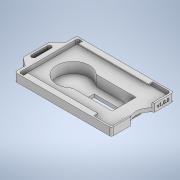
# Autodesk Inventor part: badge
Saved by Autodesk Inventor 2020 (Build 240168000, 168)
## iProperties
Created: 2019-12-22
Part Number: badge
Material: Generic
Document SubType Name: Modeling
Designer: user
Density: 1 g/cm^3
Appearance: Default
Author: user
## iProperties of the stored document _3DPrint.ipt
Created: 2019-12-23
Part Number: _3DPrint
Material: Generic
Document SubType Name: Modeling
Designer: user
Density: 1 g/cm^3
Appearance: Default
Author: user
Autodesk Inventor part; units mm, degrees
ref_plane "YZ Plane" through (0, 0, 0) normal (1, 0, 0) x (0, 1, 0)
ref_plane "XZ Plane" through (0, 0, 0) normal (0, 1, 0) x (-1, 0, 0)
ref_plane "XY Plane" through (0, 0, 0) normal (0, 0, 1) x (1, 0, 0)
sketch "Sketch1" plane through (0, 0, 0) normal (0, 1, 0) x (-1, 0, 0)
  line L0 (11.5175, 24.7666) -> (-75.997, 24.7666)
  line L1 (-76.2825, -34.0334) -> (11.5175, -34.0334)
  line L2 (13.5175, 14.7666) -> (20.6927, 9.5565)
  line L3 (21.5175, 7.9382) -> (21.5175, -15.205)
  line L4 (20.9317, -16.6192) -> (13.5175, -24.0334)
  line L5 (15.6065, 2.7666) -> (15.6065, -12.0334)
  line L6 (19.5175, -12.0334) -> (19.5175, 2.7666)
  arc A0 (17.5175, -14.0334) -> (19.5175, -12.0334) centre (17.5175, -12.0334) ccw
  arc A1 (15.6065, -12.0334) -> (17.6065, -14.0334) centre (17.6065, -12.0334) ccw
  arc A2 (17.6065, 4.7666) -> (15.6065, 2.7666) centre (17.6065, 2.7666) ccw
  arc A3 (19.5175, 2.7666) -> (17.5175, 4.7666) centre (17.5175, 2.7666) ccw
  circle A4 centre (-12.3637, -4.6334) radius 18.5
  line L7 (-63.6615, 7.6166) -> (-63.6615, -16.8834)
  line L8 (-61.6615, -18.8834) -> (-24.1615, -18.8834)
  line L9 (-24.1615, 9.6166) -> (-61.6615, 9.6166)
  arc A5 (-63.6615, -16.8834) -> (-61.6615, -18.8834) centre (-61.6615, -16.8834) ccw
  arc A6 (-61.6615, 9.6166) -> (-63.6615, 7.6166) centre (-61.6615, 7.6166) ccw
  line L10 (-28.0615, -0.3834) -> (-53.5615, -0.3834)
  line L11 (-53.5615, -0.3834) -> (-53.5615, -8.8834)
  line L12 (-53.5615, -8.8834) -> (-28.0615, -8.8834)
  line L13 (-28.0615, -8.8834) -> (-28.0615, -0.3834)
  line L14 (-77.997, 6.7666) -> (-77.997, 22.7666)
  line L15 (-78.2825, -16.0334) -> (-78.2825, -32.0334)
  line L16 (9.0144, 23.2666) -> (-74.7825, 23.2666)
  line L17 (-74.7825, -32.5334) -> (9.0144, -32.5334)
  line L18 (11.0144, -30.5334) -> (11.0144, 21.2666)
  line L19 (-76.7825, 21.2666) -> (-76.7825, 5.8175)
  line L20 (-76.7825, -30.5334) -> (-76.7825, -14.8912)
  line L21 (13.5175, 22.7666) -> (13.5175, 14.7666)
  line L22 (13.5175, -24.0334) -> (13.5175, -32.0334)
  arc A7 (-78.2825, -32.0334) -> (-76.2825, -34.0334) centre (-76.2825, -32.0334) ccw
  arc A8 (-76.7825, -30.5334) -> (-74.7825, -32.5334) centre (-74.7825, -30.5334) ccw
  arc A9 (-74.7825, 23.2666) -> (-76.7825, 21.2666) centre (-74.7825, 21.2666) ccw
  arc A10 (-75.997, 24.7666) -> (-77.997, 22.7666) centre (-75.997, 22.7666) ccw
  arc A11 (13.5175, 22.7666) -> (11.5175, 24.7666) centre (11.5175, 22.7666) ccw
  arc A12 (11.0144, 21.2666) -> (9.0144, 23.2666) centre (9.0144, 21.2666) ccw
  arc A13 (9.0144, -32.5334) -> (11.0144, -30.5334) centre (9.0144, -30.5334) ccw
  arc A14 (11.5175, -34.0334) -> (13.5175, -32.0334) centre (11.5175, -32.0334) ccw
  arc A15 (20.9317, -16.6192) -> (21.5175, -15.205) centre (19.5175, -15.205) ccw
  arc A16 (21.5175, 7.9382) -> (20.6927, 9.5565) centre (19.5175, 7.9382) ccw
  arc A17 (-78.2825, -16.0334) -> (-77.997, 6.7666) centre (-85.8517, -4.5369) ccw
  point P0 (0, 0)
  point P1 (13.5175, 24.7666)
  point P2 (-78.2825, -34.0334)
  point P3 (-77.997, 24.7666)
  point P4 (13.5175, -34.0334)
  point P5 (21.5175, -16.0334)
  point P6 (-63.6615, -18.8834)
  point P7 (17.562, 4.7661)
  point P8 (17.562, -14.0329)
  dimension "d1" = 91.8
  dimension "d2" = 8
  dimension "d11" = 10
  dimension "d12" = 10
  dimension "d14" = 2
  dimension "d16" = 2
  dimension "d17" = 2
  dimension "d19" = 18
  dimension "d20" = 37
  dimension "d24" = 39.5
  dimension "d25" = 28.5
  dimension "d26" = 2
  dimension "d28" = 10
  dimension "d32" = 10
  dimension "d33" = 10.1
  dimension "d34" = 25.5
  dimension "d36" = 1.5
  dimension "d37" = 1.5
  dimension "d40" = 1.5
  dimension "d41" = 2
  dimension "d84" = 55.8
  dimension "d85" = 10
  dimension "d86" = 10
  dimension "d87" = 27.9
  dimension "d88" = 27.9
  dimension "d89" = 18
  dimension "d104" = 87.7968
  dimension "d105" = 2.5032
  dimension "d106" = 8
  dimension "d107" = 13.65
  dimension "d108" = 13.65
  dimension "d110" = 13.7646
  constraints: 46 end point, 38 point on circle, 28 tangent, 18 centre point, 13 point on line, 12 equal radius, 7 parallel, 5 vertical, 3 horizontal, 3 perpendicular, 2 horizontal alignment, 1 collinear, 8 other
  measures "d1" distance of point (-78.282, -34.033) point (13.518, -34.033)
  measures "d2" horizontal distance of point (21.518, -16.033) L4.end
  measures "d14" distance between parallel lines of L3 L6
  measures "d16" radius of A0
  measures "d17" radius of A1
  measures "d19" distance of point (-77.997, 24.767) L14.start
  measures "d20" diameter of A4
  measures "d24" distance of point (-63.662, -18.883) L8.end
  measures "d25" distance of L8.end L9.start
  measures "d26" radius of A5
  measures "d28" distance between parallel lines of L8 L12
  measures "d32" distance between parallel lines of L10 L9
  measures "d33" distance between parallel lines of L7 L11
  measures "d34" distance of L11.end L12.end
  measures "d36" distance between parallel lines of L0 L16
  measures "d37" distance between parallel lines of L1 L17
  measures "d40" distance between parallel lines of L15 L20
  measures "d41" radius of A7
  measures "d84" distance between parallel lines of L17 L16
  measures "d85" distance of point (13.518, 24.767) L2.start
  measures "d86" distance of point (13.518, -34.033) L4.end
  measures "d87" distance from line of A4.centre L17
  measures "d88" distance from line of L16 A4.centre
  measures "d89" distance of L15.start point (-78.282, -34.033)
  measures "d104" distance between parallel lines of L19 L18
  measures "d105" distance between parallel lines of L18 L22
  measures "d106" distance between parallel lines of L21 L3
  measures "d107" distance between parallel lines of L16 L9
  measures "d108" distance between parallel lines of L17 L8
  measures "d110" radius of A17
extrude "OutsideFrame_Ex" add sketch "Sketch1" along normal blind 7.4 contours A11 L21 L2 A16 L3 A15 L4 L22 A14 L1 A7 L15 A17 L20 A8 L17 A13 L18 A12 L16 A9 L19 L14 A10 L0
extrude "CardRidge" add sketch "Sketch1" along normal blind 3.4 contours L19 A9 L16 A12 L18 A13 L17 A8 L20 A17
extrude "TokenBuffer" add sketch "Sketch1" against normal blind 9.6 contours A4 L12 L13 L10 | A4 L10 L11 L12 L8 A5 L7 A6 L9 picked at (-16.6622, -4.6334)
sketch "Sketch4" plane through (0, 0, 0) normal (0, 1, 0) x (1, 0, 0)
  arc A0 (24.1615, 18.8834) -> (24.1615, -9.6166) centre (12.3637, 4.6334) ccw projected
  circle A1 centre (12.3637, 4.6334) radius 15.5
  line L0 (23.0262, -6.6166) -> (60.6615, -6.6166)
  line L1 (60.6615, -6.6166) -> (60.6615, 15.8834)
  line L2 (60.6615, 15.8834) -> (23.0262, 15.8834)
  line L3 (23.0262, 15.8834) -> (23.0262, -6.6166)
  line L4 (61.6615, -9.6166) -> (24.1615, -9.6166) projected
  line L5 (24.1615, 18.8834) -> (61.6615, 18.8834) projected
  line L6 (63.6615, 16.8834) -> (63.6615, -7.6166) projected
  point P0 (0, 0)
  point P1 (23.0262, 15.8834)
  point P2 (23.0262, 15.8834)
  dimension "d56" = 3
  dimension "d57" = 3
  dimension "d58" = 3
  dimension "d59" = 3
  constraints: 8 end point, 2 parallel, 1 coincident, 1 horizontal, 1 perpendicular, 3 other
  measures "d57" distance between parallel lines of L4 L0
  measures "d58" distance between parallel lines of L5 L2
  measures "d59" distance between parallel lines of L6 L1
extrude "TokenCut" cut sketch "Sketch4" against normal blind 6.6
sketch "Sketch5" plane through (74.7825, 7.4, 23.2666) normal (0, 0, -1) x (-1, 0, 0)
  line L0 (-2, 0) -> (0, 0) projected
  line L1 (81.2968, 0) -> (81.2968, -1)
  line L2 (0, 0) -> (83.7968, 0) projected
  line L3 (15, 0) -> (81.2968, 0)
  line L4 (81.2968, 0) -> (81.2968, -1)
  line L5 (81.2968, -1) -> (15, -1)
  line L6 (15, -1) -> (15, 0)
  line L7 (0, -7.4) -> (0, 0) projected
  line L8 (83.7968, -7.4) -> (83.7968, 0) projected
  line L9 (0, -4) -> (83.7968, -4) projected
  point P0 (74.7825, -7.4)
  dimension "d65" = 15
  dimension "d66" = 2.5
  dimension "d67" = 1
  constraints: 10 end point, 2 parallel, 1 horizontal, 1 perpendicular, 1 point on line
  measures "d65" distance between parallel lines of L7 L6
  measures "d66" distance between parallel lines of L8 L1
  measures "d67" distance between parallel lines of L5 L2
extrude "LeftSlider" add sketch "Sketch5" along normal blind 4 contours L1 L5 L6 L2
sketch "Sketch6" plane through (-9.0144, 7.4, -32.5334) normal (0, 0, 1) x (1, 0, 0)
  line L0 (85.2968, 0) -> (-2.5032, 0) projected
  line L1 (2.5, 0) -> (68.7968, 0)
  line L2 (68.7968, 0) -> (68.7968, -1)
  line L3 (68.7968, -1) -> (2.5, -1)
  line L4 (2.5, -1) -> (2.5, 0)
  line L5 (0, -4) -> (0, 0) projected
  line L6 (83.7968, -4) -> (83.7968, 0) projected
  point P0 (9.0144, -7.4)
  point P1 (0, -7.4)
  point P2 (83.7968, -7.4)
  dimension "d71" = 2.5
  dimension "d72" = 15
  dimension "d73" = 1
  constraints: 8 end point, 2 parallel, 1 horizontal, 1 perpendicular, 1 point on line
  measures "d71" distance between parallel lines of L5 L4
  measures "d72" distance between parallel lines of L6 L2
  measures "d73" distance between parallel lines of L3 L0
extrude "RightSlider" add sketch "Sketch6" along normal blind 4
sketch "Sketch12" plane through (0, 0, 0) normal (0, 1, 0) x (1, 0, 0)
  arc A0 (23.0262, 15.8834) -> (23.0262, -6.6166) centre (12.3637, 4.6334) ccw projected
  circle A1 centre (12.3637, 4.6334) radius 15.5
  circle A2 centre (12.3637, 4.6334) radius 18.5
  line L0 (61.6615, -9.6166) -> (24.1615, -9.6166) projected
  line L1 (24.1615, -9.6166) -> (61.6615, -9.6166)
  line L2 (63.6615, 16.8834) -> (63.6615, -7.6166) projected
  arc A3 (61.6615, -9.6166) -> (63.6615, -7.6166) centre (61.6615, -7.6166) ccw
  line L3 (60.6615, -6.6166) -> (23.0262, -6.6166) projected
  line L4 (23.0262, -6.6166) -> (60.6615, -6.6166)
  line L5 (60.6615, 15.8834) -> (60.6615, -6.6166) projected
  line L6 (60.6615, -6.6166) -> (60.6615, 15.8834)
  line L7 (23.0262, 15.8834) -> (60.6615, 15.8834) projected
  line L8 (60.6615, 15.8834) -> (23.0262, 15.8834)
  line L9 (63.6615, -7.6166) -> (64.1048, 16.8834)
  line L10 (63.6615, 16.8834) -> (63.6615, -7.6166) projected
  line L11 (63.6615, -7.6166) -> (63.6615, 16.8834)
  line L12 (24.1615, 18.8834) -> (61.6615, 18.8834) projected
  arc A4 (63.6615, 16.8834) -> (61.6615, 18.8834) centre (61.6615, 16.8834) ccw
  line L13 (61.6615, 18.8834) -> (24.1615, 18.8834)
  point P0 (0, 0)
  point P1 (27.05, 15.8834)
  point P2 (27.05, -6.6166)
  constraints: 14 end point, 4 centre point, 4 point on circle, 2 coincident, 2 horizontal, 2 perpendicular, 1 collinear, 1 tangent
extrude "Extrusion13" add sketch "Sketch12" along normal blind 3.4 contours A2 L12 A4 L2 A3 L0 L3 L5 L7
extrude "Extrusion14" add sketch "Sketch12" along normal blind 3.4 contours A0 L3 A2 L7
sketch "Sketch15" plane through (78.2825, 0, -16.0334) normal (1, 0, 0) x (0, 0, -1)
  line L0 (2.191, 5.3205) -> (13.1828, 5.3205) construction
  line L1 (13.1828, 5.3205) -> (13.1828, 0.2382) construction
  line L2 (13.1828, 0.2382) -> (2.191, 0.2382) construction
  line L3 (2.191, 0.2382) -> (2.191, 5.3205) construction
  line L4 (4.2658, 4.498) -> (3.4038, 2.2107)
  line L5 (3.4038, 2.2107) -> (3.058, 2.2107)
  line L6 (3.058, 2.2107) -> (2.2033, 4.498)
  line L7 (2.2033, 4.498) -> (2.6208, 4.498)
  line L8 (2.6208, 4.498) -> (3.2457, 2.7368)
  line L9 (3.2457, 2.7368) -> (3.8657, 4.498)
  line L10 (3.8657, 4.498) -> (4.2658, 4.498)
  line L11 (6.227, 2.2107) -> (4.74, 2.2107)
  line L12 (4.74, 2.2107) -> (4.74, 2.522)
  line L13 (4.74, 2.522) -> (5.2933, 2.522)
  line L14 (5.2933, 2.522) -> (5.2933, 4.5647)
  line L15 (5.2933, 4.5647) -> (4.74, 4.5647)
  line L16 (4.74, 4.5647) -> (4.74, 4.8438)
  spline S0 degree 2 poles (4.74, 4.8438) (5.0537, 4.8438) (5.3501, 5.0216) (5.3699, 5.2686) knots 0 0 0 1 2 2 2
  line L17 (5.3699, 5.2686) -> (5.6861, 5.2686)
  line L18 (5.6861, 5.2686) -> (5.6861, 2.522)
  line L19 (5.6861, 2.522) -> (6.227, 2.522)
  line L20 (6.227, 2.522) -> (6.227, 2.2107)
  line L21 (7.4422, 2.2107) -> (6.9532, 2.2107)
  line L22 (6.9532, 2.2107) -> (6.9532, 2.7937)
  line L23 (6.9532, 2.7937) -> (7.4422, 2.7937)
  line L24 (7.4422, 2.7937) -> (7.4422, 2.2107)
  spline S1 degree 2 poles (9.9542, 3.7347) (9.9542, 2.9147) (9.4775, 2.1465) (8.9811, 2.1465) knots 0 0 0 1 2 2 2
  spline S2 degree 2 poles (8.9811, 2.1465) (8.4772, 2.1465) (8.0054, 2.9295) (8.0054, 3.7323) knots 0 0 0 1 2 2 2
  spline S3 degree 2 poles (8.0054, 3.7323) (8.0054, 4.5573) (8.4821, 5.3205) (8.9811, 5.3205) knots 0 0 0 1 2 2 2
  spline S4 degree 2 poles (8.9811, 5.3205) (9.4825, 5.3205) (9.9542, 4.5301) (9.9542, 3.7347) knots 0 0 0 1 2 2 2
  spline S5 degree 2 poles (9.4306, 2.806) (9.4899, 2.9567) (9.5393, 3.421) (9.5393, 3.7347) knots 0 0 0 1 2 2 2
  spline S6 degree 2 poles (9.5393, 3.7347) (9.5393, 4.0484) (9.4899, 4.5103) (9.4281, 4.6659) knots 0 0 0 1 2 2 2
  spline S7 degree 2 poles (9.4281, 4.6659) (9.3664, 4.8215) (9.1515, 4.9821) (8.9811, 4.9821) knots 0 0 0 1 2 2 2
  spline S8 degree 2 poles (8.9811, 4.9821) (8.8106, 4.9821) (8.5908, 4.8215) (8.5266, 4.661) knots 0 0 0 1 2 2 2
  spline S9 degree 2 poles (8.5266, 4.661) (8.4648, 4.5054) (8.4204, 4.0311) (8.4204, 3.7323) knots 0 0 0 1 2 2 2
  spline S10 degree 2 poles (8.4204, 3.7323) (8.4204, 3.4112) (8.4599, 2.9814) (8.5241, 2.8134) knots 0 0 0 1 2 2 2
  spline S11 degree 2 poles (8.5241, 2.8134) (8.5834, 2.6553) (8.8032, 2.4849) (8.9811, 2.4849) knots 0 0 0 1 2 2 2
  spline S12 degree 2 poles (8.9811, 2.4849) (9.149, 2.4849) (9.3689, 2.6455) (9.4306, 2.806) knots 0 0 0 1 2 2 2
  line L25 (10.9991, 2.2107) -> (10.51, 2.2107)
  line L26 (10.51, 2.2107) -> (10.51, 2.7937)
  line L27 (10.51, 2.7937) -> (10.9991, 2.7937)
  line L28 (10.9991, 2.7937) -> (10.9991, 2.2107)
  spline S13 degree 2 poles (13.5111, 3.7347) (13.5111, 2.9147) (13.0344, 2.1465) (12.5379, 2.1465) knots 0 0 0 1 2 2 2
  spline S14 degree 2 poles (12.5379, 2.1465) (12.034, 2.1465) (11.5622, 2.9295) (11.5622, 3.7323) knots 0 0 0 1 2 2 2
  spline S15 degree 2 poles (11.5622, 3.7323) (11.5622, 4.5573) (12.0389, 5.3205) (12.5379, 5.3205) knots 0 0 0 1 2 2 2
  spline S16 degree 2 poles (12.5379, 5.3205) (13.0393, 5.3205) (13.5111, 4.5301) (13.5111, 3.7347) knots 0 0 0 1 2 2 2
  spline S17 degree 2 poles (12.9874, 2.806) (13.0467, 2.9567) (13.0961, 3.421) (13.0961, 3.7347) knots 0 0 0 1 2 2 2
  spline S18 degree 2 poles (13.0961, 3.7347) (13.0961, 4.0484) (13.0467, 4.5103) (12.985, 4.6659) knots 0 0 0 1 2 2 2
  spline S19 degree 2 poles (12.985, 4.6659) (12.9232, 4.8215) (12.7083, 4.9821) (12.5379, 4.9821) knots 0 0 0 1 2 2 2
  spline S20 degree 2 poles (12.5379, 4.9821) (12.3675, 4.9821) (12.1476, 4.8215) (12.0834, 4.661) knots 0 0 0 1 2 2 2
  spline S21 degree 2 poles (12.0834, 4.661) (12.0217, 4.5054) (11.9772, 4.0311) (11.9772, 3.7323) knots 0 0 0 1 2 2 2
  spline S22 degree 2 poles (11.9772, 3.7323) (11.9772, 3.4112) (12.0167, 2.9814) (12.0809, 2.8134) knots 0 0 0 1 2 2 2
  spline S23 degree 2 poles (12.0809, 2.8134) (12.1402, 2.6553) (12.36, 2.4849) (12.5379, 2.4849) knots 0 0 0 1 2 2 2
  spline S24 degree 2 poles (12.5379, 2.4849) (12.7058, 2.4849) (12.9257, 2.6455) (12.9874, 2.806) knots 0 0 0 1 2 2 2
  point P0 (-16.0334, 0)
  constraints: 2 other
emboss "Emboss2" sketch "Sketch15" operation cut depth 1 direction (-1, 0, 0)
equation "\"d12\" = d11"
equation "\"d86\" = d85"
equation "\"d87\" = d88"
equation "\"d89\" = d19"
body "Solid3"
